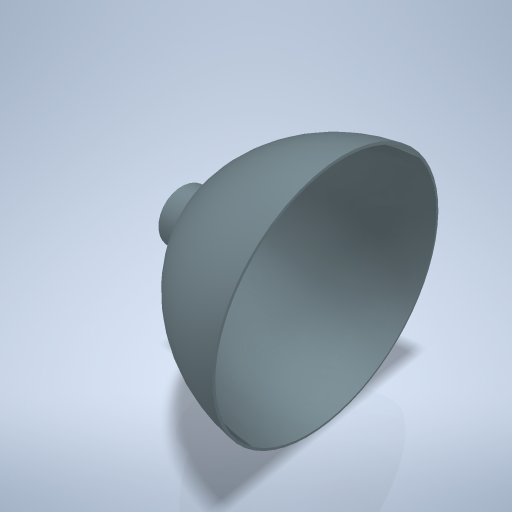
# Autodesk Inventor part: BRS_cover
Saved by Autodesk Inventor 2024.2 (Build 282272000, 272)
## iProperties
Created: 2024-05-14
Part Number: BRS_cover
Material: Blei
Document SubType Name: Modeling
Designer: Fabri
Density: 11.34 g/cm^3
Appearance: Blei
Author: Fabri
Autodesk Inventor part; units mm, degrees
ref_plane "YZ Plane" through (0, 0, 0) normal (1, 0, 0) x (0, 1, 0)
ref_plane "XZ Plane" through (0, 0, 0) normal (0, 1, 0) x (-1, 0, 0)
ref_plane "XY Plane" through (0, 0, 0) normal (0, 0, 1) x (1, 0, 0)
sketch "Skizze1" plane through (0, 0, 0) normal (0, 1, 0) x (-1, 0, 0)
  line L0 (0, 0) -> (35, 0)
  line L1 (35, 0) -> (35, 6)
  line L2 (35, 6) -> (29, 6)
  line L3 (0, 25) -> (0, 0)
  arc A0 (29, 6) -> (0, 25) centre (-0.2408, -6.9991) ccw
  dimension "d0" = 35
  dimension "d1" = 12
  dimension "d2" = 6
  dimension "d5" = 50
  dimension "d6" = 32
  constraints: 8 end point, 2 perpendicular, 2 point on circle, 1 centre point, 1 horizontal, 1 vertical
  measures "d0" distance of L0.start L0.end
  measures "d1" diameter of L1.end L0
  measures "d2" distance of L1.end L2.end
  measures "d5" diameter of L3.start L0
  measures "d6" radius of A0
revolve "Umdrehung1" add sketch "Skizze1" angle 360 about axis through (0, 0, 0) along (-1, 0, 0)
sketch "Skizze3" plane through (-35, 0, 0) normal (-1, 0, 0) x (0, 0, 1)
  circle A0 centre (0, 0) radius 6 projected
  constraints: 1 coincident
hole "Bohrung2" at (-35, 0, 0) direction (1, 0, 0) diameter 6.647 depth 6 thread size "M8x1.25" class "6H" standard "ISO Metric profile"
fillet "Rundung1" radius 2 1 edges at (-29, 0, -6)
sketch "Skizze5" plane through (0, 0, 0) normal (0, 1, 0) x (-1, 0, 0)
  arc A0 (0, -25) -> (28.4771, -7.1177) centre (-0.2408, 6.9991) ccw projected
  arc A1 (28.4771, 7.1177) -> (0, 25) centre (-0.2408, -6.9991) ccw projected
  line L0 (0, 0) -> (39.0917, 0)
  arc A2 (1, -24.4765) -> (28.0284, -6.8971) centre (-0.2408, 6.9991) ccw
  line L1 (1, -24.4765) -> (1, 0)
  line L2 (35, -6) -> (35, 6) projected
  line L3 (30.272, 6) -> (30.272, -6) projected
  line L4 (29, -3.3235) -> (35, -3.3235) projected
  arc A3 (30.272, -6) -> (28.4771, -7.1177) centre (30.272, -8) ccw projected
  line L5 (29, -3.3235) -> (29, 3.3235) projected
  arc A4 (28.0284, -6.8971) -> (29, -3.3235) centre (-11.0986, 5.66) ccw
  point P0 (29, 0)
  dimension "d25" = 1
  dimension "d26" = 0.5
  constraints: 4 end point, 4 point on circle, 2 centre point, 1 horizontal, 1 perpendicular, 1 point on line
  measures "d25" distance from line of A0.start L1
  measures "d26" radial gap between concentric circles of A0 A2
revolve "Umdrehung2" cut sketch "Skizze5" angle 360 about axis through (0, 0, 0) along (-1, 0, 0) contours L0 L5 A4 A2 L1
sketch "Skizze6" plane through (0, 0, 0) normal (1, 0, 0) x (0, 0, -1)
  circle A0 centre (0, 0) radius 25 projected
  constraints: 1 coincident
hole "Bohrung3" at (0, 0, 0) direction (-1, 0, 0) diameter 50 depth 1
